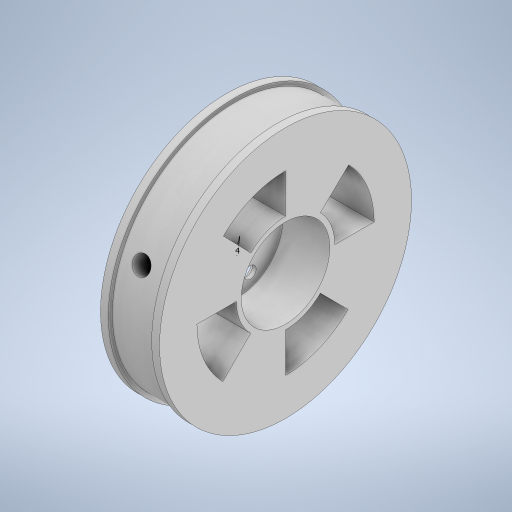
# Autodesk Inventor part: колеса прототип
Saved by Autodesk Inventor 2023 (Build 270158000, 158)
## iProperties
Created: 2026-01-23
Part Number: колеса прототип
Material: Типовые
Document SubType Name: Modeling
Designer: garin
Density: 1 g/cm^3
Appearance: По умолчанию
Author: garin
Autodesk Inventor part; units mm, degrees
ref_plane "XZ Plane" through (0, 0, 0) normal (0, 1, 0) x (-1, 0, 0)
ref_plane "XY Plane" through (0, 0, 0) normal (0, 0, 1) x (1, 0, 0)
sketch "Эскиз1" plane through (0, 0, 0) normal (1, 0, 0) x (0, 1, 0)
  circle A0 centre (0, 0) radius 33
  circle A1 centre (0, 0) radius 27.5
  line L0 (27.5, 0) -> (12.5, 0)
  line L1 (0, 27.5) -> (0, 12.5)
  arc A2 (0, -12.5) -> (12.5, 0) centre (0, 0) ccw
  arc A3 (-12.5, 0) -> (0, -12.5) centre (0, 0) ccw
  arc A4 (0, 12.5) -> (-12.5, 0) centre (0, 0) ccw
  arc A5 (12.5, 0) -> (0, 12.5) centre (0, 0) ccw
  line L2 (27.5, 0) -> (22.5, 0)
  line L3 (0, -27.5) -> (0, -22.5)
  line L4 (27.5, 0) -> (22.5, 0)
  line L5 (0, 27.5) -> (0, 22.5)
  line L6 (-27.5, 0) -> (-22.5, 0)
  circle A6 centre (0, 0) radius 22.5
  line L7 (-8.8388, -8.8388) -> (-15.9436, -15.8761)
  line L8 (-12.5, 0) -> (-22.5, 0)
  line L9 (-8.8388, 8.8388) -> (-15.8761, 15.9436)
  line L10 (8.8388, 8.8388) -> (16.0277, 15.7912)
  line L11 (12.5, 0) -> (22.5, 0)
  line L12 (0, 12.5) -> (0, 22.5)
  line L13 (8.8388, -8.8388) -> (15.7912, -16.0277)
  line L14 (0, -22.5) -> (0, -12.5)
  circle A7 centre (0, 0) radius 27.5
  circle A8 centre (0, 0) radius 32
  point P0 (-27.5, 0)
  point P1 (0, 22.5)
  point P2 (0, 22.5)
  point P3 (-22.5, 0)
  point P4 (-22.5, 0)
  dimension "d2" = 15
  dimension "d3" = 15
  dimension "d4" = 15
  dimension "d5" = 15
  dimension "d21" = 5
  dimension "d22" = 5
  dimension "d25" = 360
  dimension "d67" = 64
  constraints: 30 end point, 21 point on circle, 8 centre point, 8 coincident, 6 point on line, 5 concentric, 2 horizontal, 2 perpendicular, 1 collinear, 1 horizontal alignment, 1 vertical, 23 other
  measures "d2" distance of L0.start L0.end
  measures "d3" distance of L1.start L1.end
  measures "d4" distance of point (-27.5, 0) L8.start
  measures "d5" distance of L3.start L14.end
  measures "d21" distance of L0.start L2.end
  measures "d22" distance of L3.start L3.end
  measures "d67" diameter of A8
extrude "Выдавливание1" add sketch "Эскиз1" along normal blind 15 contours L0 A6 L1 A1 | A1 L3 A6 L0 | L1 A6 L6 A1 | A1 L6 A6 L3 | A6 L13 A2 L0 | L0 A5 L10 A6 | A6 L10 A5 L1 | L1 A4 L9 A6 | L14 A2 L13 A6 | A6 L7 A3 L14 | A2 A3 A4 A5 | L8 A3 L7 A6 | A6 L9 A4 L8 | A8
sketch "Эскиз5" plane through (15, 0, 0) normal (1, 0, 0) x (0, 0, -1)
  point P0 (0, 0)
extrude "Выдавливание3" cut sketch "Эскиз1" along normal blind 15 contours L0 A5 L10 A6 | L1 A4 L9 A6 | L14 A2 L13 A6 | L8 A3 L7 A6
sketch "Эскиз6" plane through (15, 0, 0) normal (1, 0, 0) x (0, 0, -1)
  circle A0 centre (0, 0) radius 11.25
  arc A1 (0, 12.5) -> (-8.8388, 8.8388) centre (0, 0) ccw projected
  arc A2 (0, 12.5) -> (-8.8388, 8.8388) centre (0, 0) ccw
  line L0 (0, 0) -> (-3.0615, 7.391) construction
  circle A3 centre (-3.0615, 7.391) radius 1.5
  circle A4 centre (-7.391, -3.0615) radius 1.5
  circle A5 centre (3.0615, -7.391) radius 1.5
  circle A6 centre (7.391, 3.0615) radius 1.5
  arc A7 (-3.0615, 7.391) -> (-7.391, -3.0615) centre (0, 0) ccw
  line L1 (-8.8388, 8.8388) -> (-22.3952, 22.8573) construction
  circle A8 centre (0, 0) radius 32 construction
  line L2 (-8.8388, 8.8388) -> (10.6622, 8.8388) construction
  arc A9 (-22.3952, 22.8573) -> (-32, 0) centre (0, 0) ccw construction
  line L3 (-29.5012, 12.3966) -> (-7.391, 3.0615)
  dimension "d31" = 22.5
  dimension "d72" = 8
  dimension "d74" = 3
  dimension "d77" = 360
  dimension "d79" = 134.04
  constraints: 10 point on circle, 8 centre point, 8 end point, 2 coincident, 2 concentric, 1 equal length, 1 horizontal, 9 other
  measures "d31" diameter of A0
  measures "d72" distance of L0.start L0.end
  measures "d74" diameter of A3
  measures "d79" angle of L2 L1
extrude "Выдавливание4" [suppressed]
extrude "Выдавливание5" cut sketch "Эскиз6" against normal blind 12 contours A0 | A3 | A4 | A5 | A6
extrude "Выдавливание6" [suppressed]
chamfer "Фаска2" distance 2 angle 45 1 edges at (0, -12.3912, -12.3575)
chamfer "Фаска3" distance 2 angle 45 15 edges at (0, -20.7964, -8.5883) (0, -17.5, 0) (0, -11.5485, -4.7835) (0, 0, -17.5) (0, 8.5331, -20.8191) (0, 12.315, -12.4333) (0, 4.7835, -11.5485) (0, 17.5, 0) (0, 11.5485, 4.7835) (0, 20.8191, 8.5331) (0, 12.4333, 12.315) (0, 0, 17.5) (0, -4.7835, 11.5485) (0, -12.3575, 12.3912) (0, -8.5883, 20.7964)
ref_plane "РабПлоскость3" through (2, 0, 0) normal (1, 0, 0) x (0, 1, 0)
sketch "Эскиз10" plane through (2, 0, 0) normal (1, 0, 0) x (0, 1, 0)
  circle A0 centre (0, 0) radius 26.5
  circle A1 centre (0, 0) radius 27.5 projected
  circle A2 centre (0, 0) radius 26.5
  dimension "d66" = 53
  constraints: 2 centre point, 2 coincident, 1 concentric
  measures "d66" diameter of A0
sketch "Эскиз11" plane through (0, 0, 0) normal (-1, 0, 0) x (0, 0, 1)
  circle A0 centre (0, 0) radius 31
  circle A1 centre (0, 0) radius 32
  dimension "d68" = 62
  constraints: 2 centre point, 2 coincident
  measures "d68" diameter of A0
extrude "Выдавливание9" cut sketch "Эскиз11" against normal blind 11 from surface at -2
extrude "Выдавливание10" cut sketch "Эскиз6" against normal blind 15 contours A3 | A5
chamfer "Фаска4" distance 2 angle 45 2 edges at (0, 7.391, 4.5615) (0, -7.391, -1.5615)
sketch "Эскиз12" plane through (15, 0, 0) normal (1, 0, 0) x (0, 0, -1)
  circle A0 centre (0, 0) radius 32 projected
  arc A1 (0, 12.5) -> (-8.8388, 8.8388) centre (0, 0) ccw projected
  line L0 (-8.8388, 8.8388) -> (-22.3952, 22.8573)
  circle A2 centre (0, 0) radius 32 projected
  line L1 (-8.8388, 8.8388) -> (10.6622, 8.8388) construction
  point P0 (0, 0)
  point P1 (-32, 0)
  dimension "d85" = 134.04
  constraints: 4 end point, 1 coincident, 1 equal length, 1 horizontal, 1 horizontal alignment, 1 point on circle, 1 other
  measures "d85" angle of L1 L0
ref_plane "РабПлоскость4" through (15, 12.3966, 29.5012) normal (0, 0.387395, 0.9219138) x (-1, 0, 0)
sketch "Эскиз14" plane through (15, 12.3966, 29.5012) normal (0, 0.387395, 0.9219138) x (-1, 0, 0)
  circle A0 centre (8, 0) radius 2.25
  point P0 (15, 0)
  dimension "d87" = 4.5
  constraints: 1 centre point, 1 coincident
  measures "d87" diameter of A0
extrude "Выдавливание11" cut sketch "Эскиз14" against normal blind 25
sketch "Эскиз15" plane through (3, 0, 0) normal (1, 0, 0) x (0, 0, -1)
  circle A0 centre (0, 0) radius 2
  dimension "d90" = 4
  constraints: 1 centre point, 1 coincident
  measures "d90" diameter of A0
